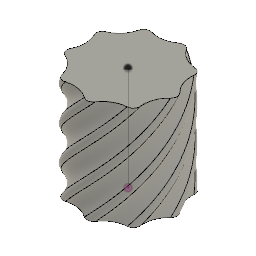
Calibration Set (Autodesk Fusion 360 design; units mm, degrees)
Autodesk Fusion 360 part; units mm, degrees
sketch "Base Profile" plane through (0, 0, 0) normal (0, 0, 1) x (1, 0, 0)
  arc A0 (-5.6274, 12.5123) -> (-8.0222, 11.1296) centre (-6.1732, 10.6923) ccw
  arc A1 (-5.6274, 12.5123) -> (1.0086, 13.6824) centre (-3.473, 19.6962) ccw
  arc A2 (3.7319, 13.2022) -> (1.0086, 13.6824) centre (2.1439, 12.1589) ccw
  arc A3 (3.7319, 13.2022) -> (9.5675, 9.833) centre (10, 17.3205) ccw
  arc A4 (11.345, 7.7147) -> (9.5675, 9.833) centre (9.4579, 7.9362) ccw
  arc A5 (11.345, 7.7147) -> (13.6497, 1.3826) centre (18.7939, 6.8404) ccw
  arc A6 (13.6497, -1.3826) -> (13.6497, 1.3826) centre (12.3465, 0) ccw
  arc A7 (13.6497, -1.3826) -> (11.345, -7.7147) centre (18.7939, -6.8404) ccw
  arc A8 (9.5675, -9.833) -> (11.345, -7.7147) centre (9.4579, -7.9362) ccw
  arc A9 (9.5675, -9.833) -> (3.7319, -13.2022) centre (10, -17.3205) ccw
  arc A10 (1.0086, -13.6824) -> (3.7319, -13.2022) centre (2.1439, -12.1589) ccw
  arc A11 (1.0086, -13.6824) -> (-5.6274, -12.5123) centre (-3.473, -19.6962) ccw
  arc A12 (-8.0222, -11.1296) -> (-5.6274, -12.5123) centre (-6.1732, -10.6923) ccw
  arc A13 (-8.0222, -11.1296) -> (-12.3536, -5.9677) centre (-15.3209, -12.8558) ccw
  arc A14 (-13.2994, -3.3692) -> (-12.3536, -5.9677) centre (-11.6019, -4.2227) ccw
  arc A15 (-13.2994, -3.3692) -> (-13.2994, 3.3692) centre (-20, 0) ccw
  arc A16 (-12.3536, 5.9677) -> (-13.2994, 3.3692) centre (-11.6019, 4.2227) ccw
  arc A17 (-12.3536, 5.9677) -> (-8.0222, 11.1296) centre (-15.3209, 12.8558) ccw
  dimension "d1" = 1.9
  measures "d1" radius of A0
sketch "+0.6" plane through (0, 0, 0) normal (0, 0, 1) x (1, 0, 0)
  arc A0 (-5.6274, 12.5123) -> (-8.0222, 11.1296) centre (-6.1732, 10.6923) ccw
  arc A1 (-5.6274, 12.5123) -> (1.0086, 13.6824) centre (-3.473, 19.6962) ccw
  arc A2 (3.7319, 13.2022) -> (1.0086, 13.6824) centre (2.1439, 12.1589) ccw
  arc A3 (3.7319, 13.2022) -> (9.5675, 9.833) centre (10, 17.3205) ccw
  arc A4 (11.345, 7.7147) -> (9.5675, 9.833) centre (9.4579, 7.9362) ccw
  arc A5 (11.345, 7.7147) -> (13.6497, 1.3826) centre (18.7939, 6.8404) ccw
  arc A6 (13.6497, -1.3826) -> (13.6497, 1.3826) centre (12.3465, 0) ccw
  arc A7 (13.6497, -1.3826) -> (11.345, -7.7147) centre (18.7939, -6.8404) ccw
  arc A8 (9.5675, -9.833) -> (11.345, -7.7147) centre (9.4579, -7.9362) ccw
  arc A9 (9.5675, -9.833) -> (3.7319, -13.2022) centre (10, -17.3205) ccw
  arc A10 (1.0086, -13.6824) -> (3.7319, -13.2022) centre (2.1439, -12.1589) ccw
  arc A11 (1.0086, -13.6824) -> (-5.6274, -12.5123) centre (-3.473, -19.6962) ccw
  arc A12 (-8.0222, -11.1296) -> (-5.6274, -12.5123) centre (-6.1732, -10.6923) ccw
  arc A13 (-8.0222, -11.1296) -> (-12.3536, -5.9677) centre (-15.3209, -12.8558) ccw
  arc A14 (-13.2994, -3.3692) -> (-12.3536, -5.9677) centre (-11.6019, -4.2227) ccw
  arc A15 (-13.2994, -3.3692) -> (-13.2994, 3.3692) centre (-20, 0) ccw
  arc A16 (-12.3536, 5.9677) -> (-13.2994, 3.3692) centre (-11.6019, 4.2227) ccw
  arc A17 (-12.3536, 5.9677) -> (-8.0222, 11.1296) centre (-15.3209, 12.8558) ccw
  arc A18 (11.9409, 7.6447) -> (9.6021, 10.432) centre (9.4579, 7.9362) ccw
  arc A19 (4.2333, 13.5317) -> (9.6021, 10.432) centre (10, 17.3205) ccw
  arc A20 (4.2333, 13.5317) -> (0.6501, 14.1635) centre (2.1439, 12.1589) ccw
  arc A21 (-5.4551, 13.087) -> (0.6501, 14.1635) centre (-3.473, 19.6962) ccw
  arc A22 (-5.4551, 13.087) -> (-8.6061, 11.2677) centre (-6.1732, 10.6923) ccw
  arc A23 (-12.591, 6.5188) -> (-8.6061, 11.2677) centre (-15.3209, 12.8558) ccw
  arc A24 (-12.591, 6.5188) -> (-13.8354, 3.0997) centre (-11.6019, 4.2227) ccw
  arc A25 (-13.8354, -3.0997) -> (-13.8354, 3.0997) centre (-20, 0) ccw
  arc A26 (-13.8354, -3.0997) -> (-12.591, -6.5188) centre (-11.6019, -4.2227) ccw
  arc A27 (-8.6061, -11.2677) -> (-12.591, -6.5188) centre (-15.3209, -12.8558) ccw
  arc A28 (-8.6061, -11.2677) -> (-5.4551, -13.087) centre (-6.1732, -10.6923) ccw
  arc A29 (0.6501, -14.1635) -> (-5.4551, -13.087) centre (-3.473, -19.6962) ccw
  arc A30 (0.6501, -14.1635) -> (4.2333, -13.5317) centre (2.1439, -12.1589) ccw
  arc A31 (9.6021, -10.432) -> (4.2333, -13.5317) centre (10, -17.3205) ccw
  arc A32 (9.6021, -10.432) -> (11.9409, -7.6447) centre (9.4579, -7.9362) ccw
  arc A33 (14.0612, -1.8193) -> (11.9409, -7.6447) centre (18.7939, -6.8404) ccw
  arc A34 (14.0612, -1.8193) -> (14.0612, 1.8193) centre (12.3465, 0) ccw
  arc A35 (11.9409, 7.6447) -> (14.0612, 1.8193) centre (18.7939, 6.8404) ccw
  dimension "d2" = 1.9
  dimension "d3" = 0.6
  measures "d2" radius of A0
sketch "+0.7" plane through (0, 0, 0) normal (0, 0, 1) x (1, 0, 0)
  arc A0 (-5.6274, 12.5123) -> (-8.0222, 11.1296) centre (-6.1732, 10.6923) ccw
  arc A1 (-5.6274, 12.5123) -> (1.0086, 13.6824) centre (-3.473, 19.6962) ccw
  arc A2 (3.7319, 13.2022) -> (1.0086, 13.6824) centre (2.1439, 12.1589) ccw
  arc A3 (3.7319, 13.2022) -> (9.5675, 9.833) centre (10, 17.3205) ccw
  arc A4 (11.345, 7.7147) -> (9.5675, 9.833) centre (9.4579, 7.9362) ccw
  arc A5 (11.345, 7.7147) -> (13.6497, 1.3826) centre (18.7939, 6.8404) ccw
  arc A6 (13.6497, -1.3826) -> (13.6497, 1.3826) centre (12.3465, 0) ccw
  arc A7 (13.6497, -1.3826) -> (11.345, -7.7147) centre (18.7939, -6.8404) ccw
  arc A8 (9.5675, -9.833) -> (11.345, -7.7147) centre (9.4579, -7.9362) ccw
  arc A9 (9.5675, -9.833) -> (3.7319, -13.2022) centre (10, -17.3205) ccw
  arc A10 (1.0086, -13.6824) -> (3.7319, -13.2022) centre (2.1439, -12.1589) ccw
  arc A11 (1.0086, -13.6824) -> (-5.6274, -12.5123) centre (-3.473, -19.6962) ccw
  arc A12 (-8.0222, -11.1296) -> (-5.6274, -12.5123) centre (-6.1732, -10.6923) ccw
  arc A13 (-8.0222, -11.1296) -> (-12.3536, -5.9677) centre (-15.3209, -12.8558) ccw
  arc A14 (-13.2994, -3.3692) -> (-12.3536, -5.9677) centre (-11.6019, -4.2227) ccw
  arc A15 (-13.2994, -3.3692) -> (-13.2994, 3.3692) centre (-20, 0) ccw
  arc A16 (-12.3536, 5.9677) -> (-13.2994, 3.3692) centre (-11.6019, 4.2227) ccw
  arc A17 (-12.3536, 5.9677) -> (-8.0222, 11.1296) centre (-15.3209, 12.8558) ccw
  arc A18 (12.0402, 7.6331) -> (9.6079, 10.5318) centre (9.4579, 7.9362) ccw
  arc A19 (4.3169, 13.5866) -> (9.6079, 10.5318) centre (10, 17.3205) ccw
  arc A20 (4.3169, 13.5866) -> (0.5903, 14.2437) centre (2.1439, 12.1589) ccw
  arc A21 (-5.4263, 13.1828) -> (0.5903, 14.2437) centre (-3.473, 19.6962) ccw
  arc A22 (-5.4263, 13.1828) -> (-8.7034, 11.2907) centre (-6.1732, 10.6923) ccw
  arc A23 (-12.6305, 6.6106) -> (-8.7034, 11.2907) centre (-15.3209, 12.8558) ccw
  arc A24 (-12.6305, 6.6106) -> (-13.9248, 3.0547) centre (-11.6019, 4.2227) ccw
  arc A25 (-13.9248, -3.0547) -> (-13.9248, 3.0547) centre (-20, 0) ccw
  arc A26 (-13.9248, -3.0547) -> (-12.6305, -6.6106) centre (-11.6019, -4.2227) ccw
  arc A27 (-8.7034, -11.2907) -> (-12.6305, -6.6106) centre (-15.3209, -12.8558) ccw
  arc A28 (-8.7034, -11.2907) -> (-5.4263, -13.1828) centre (-6.1732, -10.6923) ccw
  arc A29 (0.5903, -14.2437) -> (-5.4263, -13.1828) centre (-3.473, -19.6962) ccw
  arc A30 (0.5903, -14.2437) -> (4.3169, -13.5866) centre (2.1439, -12.1589) ccw
  arc A31 (9.6079, -10.5318) -> (4.3169, -13.5866) centre (10, -17.3205) ccw
  arc A32 (9.6079, -10.5318) -> (12.0402, -7.6331) centre (9.4579, -7.9362) ccw
  arc A33 (14.1298, -1.892) -> (12.0402, -7.6331) centre (18.7939, -6.8404) ccw
  arc A34 (14.1298, -1.892) -> (14.1298, 1.892) centre (12.3465, 0) ccw
  arc A35 (12.0402, 7.6331) -> (14.1298, 1.892) centre (18.7939, 6.8404) ccw
  dimension "d4" = 1.9
  dimension "d5" = 0.7
  measures "d4" radius of A0
sketch "+0.8" plane through (0, 0, 0) normal (0, 0, 1) x (1, 0, 0)
  arc A0 (-5.6274, 12.5123) -> (-8.0222, 11.1296) centre (-6.1732, 10.6923) ccw
  arc A1 (-5.6274, 12.5123) -> (1.0086, 13.6824) centre (-3.473, 19.6962) ccw
  arc A2 (3.7319, 13.2022) -> (1.0086, 13.6824) centre (2.1439, 12.1589) ccw
  arc A3 (3.7319, 13.2022) -> (9.5675, 9.833) centre (10, 17.3205) ccw
  arc A4 (11.345, 7.7147) -> (9.5675, 9.833) centre (9.4579, 7.9362) ccw
  arc A5 (11.345, 7.7147) -> (13.6497, 1.3826) centre (18.7939, 6.8404) ccw
  arc A6 (13.6497, -1.3826) -> (13.6497, 1.3826) centre (12.3465, 0) ccw
  arc A7 (13.6497, -1.3826) -> (11.345, -7.7147) centre (18.7939, -6.8404) ccw
  arc A8 (9.5675, -9.833) -> (11.345, -7.7147) centre (9.4579, -7.9362) ccw
  arc A9 (9.5675, -9.833) -> (3.7319, -13.2022) centre (10, -17.3205) ccw
  arc A10 (1.0086, -13.6824) -> (3.7319, -13.2022) centre (2.1439, -12.1589) ccw
  arc A11 (1.0086, -13.6824) -> (-5.6274, -12.5123) centre (-3.473, -19.6962) ccw
  arc A12 (-8.0222, -11.1296) -> (-5.6274, -12.5123) centre (-6.1732, -10.6923) ccw
  arc A13 (-8.0222, -11.1296) -> (-12.3536, -5.9677) centre (-15.3209, -12.8558) ccw
  arc A14 (-13.2994, -3.3692) -> (-12.3536, -5.9677) centre (-11.6019, -4.2227) ccw
  arc A15 (-13.2994, -3.3692) -> (-13.2994, 3.3692) centre (-20, 0) ccw
  arc A16 (-12.3536, 5.9677) -> (-13.2994, 3.3692) centre (-11.6019, 4.2227) ccw
  arc A17 (-12.3536, 5.9677) -> (-8.0222, 11.1296) centre (-15.3209, 12.8558) ccw
  arc A18 (4.4005, 13.6415) -> (9.6136, 10.6317) centre (10, 17.3205) ccw
  arc A19 (12.1395, 7.6214) -> (9.6136, 10.6317) centre (9.4579, 7.9362) ccw
  arc A20 (12.1395, 7.6214) -> (14.1984, 1.9648) centre (18.7939, 6.8404) ccw
  arc A21 (14.1984, -1.9648) -> (14.1984, 1.9648) centre (12.3465, 0) ccw
  arc A22 (14.1984, -1.9648) -> (12.1395, -7.6214) centre (18.7939, -6.8404) ccw
  arc A23 (9.6136, -10.6317) -> (12.1395, -7.6214) centre (9.4579, -7.9362) ccw
  arc A24 (9.6136, -10.6317) -> (4.4005, -13.6415) centre (10, -17.3205) ccw
  arc A25 (0.5306, -14.3238) -> (4.4005, -13.6415) centre (2.1439, -12.1589) ccw
  arc A26 (0.5306, -14.3238) -> (-5.3976, -13.2785) centre (-3.473, -19.6962) ccw
  arc A27 (-8.8007, -11.3138) -> (-5.3976, -13.2785) centre (-6.1732, -10.6923) ccw
  arc A28 (-8.8007, -11.3138) -> (-12.6701, -6.7024) centre (-15.3209, -12.8558) ccw
  arc A29 (-14.0141, -3.0098) -> (-12.6701, -6.7024) centre (-11.6019, -4.2227) ccw
  arc A30 (-14.0141, -3.0098) -> (-14.0141, 3.0098) centre (-20, 0) ccw
  arc A31 (-12.6701, 6.7024) -> (-14.0141, 3.0098) centre (-11.6019, 4.2227) ccw
  arc A32 (-12.6701, 6.7024) -> (-8.8007, 11.3138) centre (-15.3209, 12.8558) ccw
  arc A33 (-5.3976, 13.2785) -> (-8.8007, 11.3138) centre (-6.1732, 10.6923) ccw
  arc A34 (-5.3976, 13.2785) -> (0.5306, 14.3238) centre (-3.473, 19.6962) ccw
  arc A35 (4.4005, 13.6415) -> (0.5306, 14.3238) centre (2.1439, 12.1589) ccw
  dimension "d6" = 1.9
  dimension "d7" = 0.8
  measures "d6" radius of A0
sketch "-1.0" plane through (0, 0, 0) normal (0, 0, 1) x (1, 0, 0)
  arc A0 (-5.6274, 12.5123) -> (-8.0222, 11.1296) centre (-6.1732, 10.6923) ccw
  arc A1 (-5.6274, 12.5123) -> (1.0086, 13.6824) centre (-3.473, 19.6962) ccw
  arc A2 (3.7319, 13.2022) -> (1.0086, 13.6824) centre (2.1439, 12.1589) ccw
  arc A3 (3.7319, 13.2022) -> (9.5675, 9.833) centre (10, 17.3205) ccw
  arc A4 (11.345, 7.7147) -> (9.5675, 9.833) centre (9.4579, 7.9362) ccw
  arc A5 (11.345, 7.7147) -> (13.6497, 1.3826) centre (18.7939, 6.8404) ccw
  arc A6 (13.6497, -1.3826) -> (13.6497, 1.3826) centre (12.3465, 0) ccw
  arc A7 (13.6497, -1.3826) -> (11.345, -7.7147) centre (18.7939, -6.8404) ccw
  arc A8 (9.5675, -9.833) -> (11.345, -7.7147) centre (9.4579, -7.9362) ccw
  arc A9 (9.5675, -9.833) -> (3.7319, -13.2022) centre (10, -17.3205) ccw
  arc A10 (1.0086, -13.6824) -> (3.7319, -13.2022) centre (2.1439, -12.1589) ccw
  arc A11 (1.0086, -13.6824) -> (-5.6274, -12.5123) centre (-3.473, -19.6962) ccw
  arc A12 (-8.0222, -11.1296) -> (-5.6274, -12.5123) centre (-6.1732, -10.6923) ccw
  arc A13 (-8.0222, -11.1296) -> (-12.3536, -5.9677) centre (-15.3209, -12.8558) ccw
  arc A14 (-13.2994, -3.3692) -> (-12.3536, -5.9677) centre (-11.6019, -4.2227) ccw
  arc A15 (-13.2994, -3.3692) -> (-13.2994, 3.3692) centre (-20, 0) ccw
  arc A16 (-12.3536, 5.9677) -> (-13.2994, 3.3692) centre (-11.6019, 4.2227) ccw
  arc A17 (-12.3536, 5.9677) -> (-8.0222, 11.1296) centre (-15.3209, 12.8558) ccw
  arc A18 (10.3518, 7.8312) -> (9.5098, 8.8347) centre (9.4579, 7.9362) ccw
  arc A19 (2.8961, 12.6531) -> (9.5098, 8.8347) centre (10, 17.3205) ccw
  arc A20 (2.8961, 12.6531) -> (1.6062, 12.8805) centre (2.1439, 12.1589) ccw
  arc A21 (-5.9147, 11.5544) -> (1.6062, 12.8805) centre (-3.473, 19.6962) ccw
  arc A22 (-5.9147, 11.5544) -> (-7.0491, 10.8995) centre (-6.1732, 10.6923) ccw
  arc A23 (-11.958, 5.0493) -> (-7.0491, 10.8995) centre (-15.3209, 12.8558) ccw
  arc A24 (-11.958, 5.0493) -> (-12.406, 3.8184) centre (-11.6019, 4.2227) ccw
  arc A25 (-12.406, -3.8184) -> (-12.406, 3.8184) centre (-20, 0) ccw
  arc A26 (-12.406, -3.8184) -> (-11.958, -5.0493) centre (-11.6019, -4.2227) ccw
  arc A27 (-7.0491, -10.8995) -> (-11.958, -5.0493) centre (-15.3209, -12.8558) ccw
  arc A28 (-7.0491, -10.8995) -> (-5.9147, -11.5544) centre (-6.1732, -10.6923) ccw
  arc A29 (1.6062, -12.8805) -> (-5.9147, -11.5544) centre (-3.473, -19.6962) ccw
  arc A30 (1.6062, -12.8805) -> (2.8961, -12.6531) centre (2.1439, -12.1589) ccw
  arc A31 (9.5098, -8.8347) -> (2.8961, -12.6531) centre (10, -17.3205) ccw
  arc A32 (9.5098, -8.8347) -> (10.3518, -7.8312) centre (9.4579, -7.9362) ccw
  arc A33 (12.9638, -0.6549) -> (10.3518, -7.8312) centre (18.7939, -6.8404) ccw
  arc A34 (12.9638, -0.6549) -> (12.9638, 0.6549) centre (12.3465, 0) ccw
  arc A35 (10.3518, 7.8312) -> (12.9638, 0.6549) centre (18.7939, 6.8404) ccw
  dimension "d8" = 1.9
  dimension "d9" = 1
  measures "d8" radius of A0
sketch "-1.5" plane through (0, 0, 0) normal (0, 0, 1) x (1, 0, 0)
  arc A0 (-5.6274, 12.5123) -> (-8.0222, 11.1296) centre (-6.1732, 10.6923) ccw
  arc A1 (-5.6274, 12.5123) -> (1.0086, 13.6824) centre (-3.473, 19.6962) ccw
  arc A2 (3.7319, 13.2022) -> (1.0086, 13.6824) centre (2.1439, 12.1589) ccw
  arc A3 (3.7319, 13.2022) -> (9.5675, 9.833) centre (10, 17.3205) ccw
  arc A4 (11.345, 7.7147) -> (9.5675, 9.833) centre (9.4579, 7.9362) ccw
  arc A5 (11.345, 7.7147) -> (13.6497, 1.3826) centre (18.7939, 6.8404) ccw
  arc A6 (13.6497, -1.3826) -> (13.6497, 1.3826) centre (12.3465, 0) ccw
  arc A7 (13.6497, -1.3826) -> (11.345, -7.7147) centre (18.7939, -6.8404) ccw
  arc A8 (9.5675, -9.833) -> (11.345, -7.7147) centre (9.4579, -7.9362) ccw
  arc A9 (9.5675, -9.833) -> (3.7319, -13.2022) centre (10, -17.3205) ccw
  arc A10 (1.0086, -13.6824) -> (3.7319, -13.2022) centre (2.1439, -12.1589) ccw
  arc A11 (1.0086, -13.6824) -> (-5.6274, -12.5123) centre (-3.473, -19.6962) ccw
  arc A12 (-8.0222, -11.1296) -> (-5.6274, -12.5123) centre (-6.1732, -10.6923) ccw
  arc A13 (-8.0222, -11.1296) -> (-12.3536, -5.9677) centre (-15.3209, -12.8558) ccw
  arc A14 (-13.2994, -3.3692) -> (-12.3536, -5.9677) centre (-11.6019, -4.2227) ccw
  arc A15 (-13.2994, -3.3692) -> (-13.2994, 3.3692) centre (-20, 0) ccw
  arc A16 (-12.3536, 5.9677) -> (-13.2994, 3.3692) centre (-11.6019, 4.2227) ccw
  arc A17 (-12.3536, 5.9677) -> (-8.0222, 11.1296) centre (-15.3209, 12.8558) ccw
  arc A18 (12.6208, -0.2911) -> (12.6208, 0.2911) centre (12.3465, 0) ccw
  arc A19 (9.8552, 7.8895) -> (12.6208, 0.2911) centre (18.7939, 6.8404) ccw
  arc A20 (9.8552, 7.8895) -> (9.481, 8.3355) centre (9.4579, 7.9362) ccw
  arc A21 (2.4782, 12.3785) -> (9.481, 8.3355) centre (10, 17.3205) ccw
  arc A22 (2.4782, 12.3785) -> (1.9049, 12.4796) centre (2.1439, 12.1589) ccw
  arc A23 (-6.0583, 11.0755) -> (1.9049, 12.4796) centre (-3.473, 19.6962) ccw
  arc A24 (-6.0583, 11.0755) -> (-6.5625, 10.7844) centre (-6.1732, 10.6923) ccw
  arc A25 (-11.7601, 4.5901) -> (-6.5625, 10.7844) centre (-15.3209, 12.8558) ccw
  arc A26 (-11.7601, 4.5901) -> (-11.9592, 4.043) centre (-11.6019, 4.2227) ccw
  arc A27 (-11.9592, -4.043) -> (-11.9592, 4.043) centre (-20, 0) ccw
  arc A28 (-11.9592, -4.043) -> (-11.7601, -4.5901) centre (-11.6019, -4.2227) ccw
  arc A29 (-6.5625, -10.7844) -> (-11.7601, -4.5901) centre (-15.3209, -12.8558) ccw
  arc A30 (-6.5625, -10.7844) -> (-6.0583, -11.0755) centre (-6.1732, -10.6923) ccw
  arc A31 (1.9049, -12.4796) -> (-6.0583, -11.0755) centre (-3.473, -19.6962) ccw
  arc A32 (1.9049, -12.4796) -> (2.4782, -12.3785) centre (2.1439, -12.1589) ccw
  arc A33 (9.481, -8.3355) -> (2.4782, -12.3785) centre (10, -17.3205) ccw
  arc A34 (9.481, -8.3355) -> (9.8552, -7.8895) centre (9.4579, -7.9362) ccw
  arc A35 (12.6208, -0.2911) -> (9.8552, -7.8895) centre (18.7939, -6.8404) ccw
  dimension "d10" = 1.9
  dimension "d11" = 1.5
  measures "d10" radius of A0
sketch "Upright Path" plane through (0, 0, 0) normal (1, 0, 0) x (0, 1, 0)
  line L0 (0, 0) -> (0, 30)
  dimension "d12" = 30
sweep "Sweep1" add twist angle 120 profiles "Base Profile" path "Upright Path" along L0 section 1 makes body 1
sweep "Sweep2" add twist angle 120 profiles "-1.0" path "Upright Path" along L0 section 1 separate body makes body 2
sweep "Sweep3" add twist angle 120 profiles "-1.5" path "Upright Path" along L0 section 1 separate body makes body 3
sweep "Sweep4" add twist angle 120 profiles "+0.6" path "Upright Path" along L0 section 1 contours A0 A1 A2 A3 A4 A5 A6 A7 A8 A9 A10 A11 A12 A13 A14 A15 A16 A17 | A18 A19 A20 A21 A22 A23 A24 A25 A26 A27 A28 A29 A30 A31 A32 A33 A34 A35 separate body makes body 4
sweep "Sweep5" add twist angle 120 profiles "+0.7" path "Upright Path" along L0 section 1 contours A0 A1 A2 A3 A4 A5 A6 A7 A8 A9 A10 A11 A12 A13 A14 A15 A16 A17 | A18 A19 A20 A21 A22 A23 A24 A25 A26 A27 A28 A29 A30 A31 A32 A33 A34 A35 separate body makes body 5
sweep "Sweep6" add twist angle 120 profiles "+0.8" path "Upright Path" along L0 section 1 contours A0 A1 A2 A3 A4 A5 A6 A7 A8 A9 A10 A11 A12 A13 A14 A15 A16 A17 | A18 A19 A20 A21 A22 A23 A24 A25 A26 A27 A28 A29 A30 A31 A32 A33 A34 A35 separate body makes body 6
hidden bodies 2 3 4 5 6
named bodies: "Solid/Vase", "1mm Wall", "1.5mm Wall", "+0.6 Vase", "+0.7 Vase", "+0.8 Vase"
